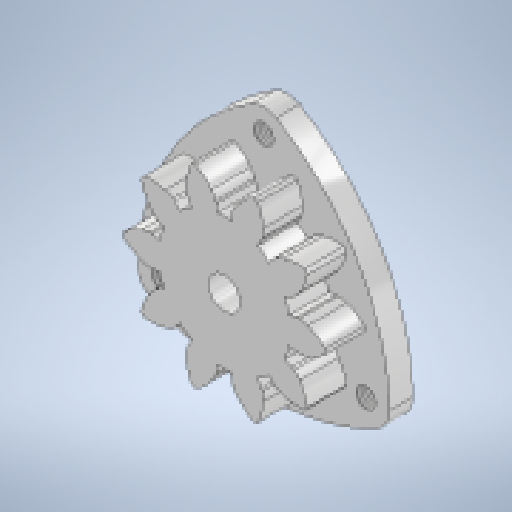
# Autodesk Inventor part: 多段ギアm2z10t8
Saved by Autodesk Inventor 2023 (Build 270158030, 158C)
## iProperties
Created: 2022-01-10
Part Number: 多段ギアm2z10t8
Material: アルミニウム 2014-T6
Document SubType Name: Modeling
Designer: acps
Density: 2.78927 g/cm^3
Appearance: サテン
Mass: 10.7159 g
Surface Area: 25.2572 cm^2
Volume: 3.84181 cm^3
Author: acps
Autodesk Inventor part; units mm, degrees
ref_plane "YZ Plane" through (0, 0, 0) normal (1, 0, 0) x (0, 1, 0)
ref_plane "XZ Plane" through (0, 0, 0) normal (0, 1, 0) x (-1, 0, 0)
ref_plane "XY Plane" through (0, 0, 0) normal (0, 0, 1) x (1, 0, 0)
sketch "Sketch1" plane through (0, 0, 0) normal (0, 0, 1) x (1, 0, 0)
  line L0 (0, -14) -> (0, 14)
  arc A0 (1.1104, 9.6344) -> (1.0261, 9.3407) centre (2.3502, 9.1195) ccw
  arc A1 (1.6598, 10.577) -> (1.1104, 9.6344) centre (4.6214, 8.2197) ccw
  arc A2 (3.6803, 12.3001) -> (1.6598, 10.577) centre (7.0807, 6.2665) ccw
  arc A3 (-4.7646, 8.4471) -> (-4.6602, 8.16) centre (-3.4589, 8.7593) ccw
  arc A4 (-4.8742, 9.5326) -> (-4.7646, 8.4471) centre (-1.0926, 9.3663) ccw
  arc A5 (-4.2524, 12.1142) -> (-4.8742, 9.5326) centre (2.0451, 9.2317) ccw
  arc A6 (-8.8197, 4.0333) -> (-8.5665, 3.8624) centre (-7.9469, 5.0533) ccw
  arc A7 (-9.5464, 4.847) -> (-8.8197, 4.0333) centre (-6.3893, 6.9353) ccw
  arc A8 (-10.5608, 7.3011) -> (-9.5464, 4.847) centre (-3.7717, 8.6706) ccw
  arc A9 (-9.506, -1.9211) -> (-9.2007, -1.9105) centre (-9.3994, -0.5829) ccw
  arc A10 (-10.5722, -1.6899) -> (-9.506, -1.9211) centre (-9.2455, 1.8552) ccw
  arc A11 (-12.8353, -0.3008) -> (-10.5722, -1.6899) centre (-8.1479, 4.7977) ccw
  arc A12 (-6.5613, -7.1417) -> (-6.3205, -6.9537) centre (-7.2617, -5.9964) ccw
  arc A13 (-7.5598, -7.5814) -> (-6.5613, -7.1417) centre (-8.5702, -3.9334) ccw
  arc A14 (-10.2072, -7.7878) -> (-7.5598, -7.5814) centre (-9.4118, -0.9078) ccw
  arc A15 (-1.1104, -9.6344) -> (-1.0261, -9.3407) centre (-2.3502, -9.1195) ccw
  arc A16 (-1.6598, -10.577) -> (-1.1104, -9.6344) centre (-4.6214, -8.2197) ccw
  arc A17 (-3.6803, -12.3001) -> (-1.6598, -10.577) centre (-7.0807, -6.2665) ccw
  arc A18 (4.7646, -8.4471) -> (4.6602, -8.16) centre (3.4589, -8.7593) ccw
  arc A19 (4.8742, -9.5326) -> (4.7646, -8.4471) centre (1.0926, -9.3663) ccw
  arc A20 (4.2524, -12.1142) -> (4.8742, -9.5326) centre (-2.0451, -9.2317) ccw
  arc A21 (8.8197, -4.0333) -> (8.5665, -3.8624) centre (7.9469, -5.0533) ccw
  arc A22 (9.5464, -4.847) -> (8.8197, -4.0333) centre (6.3893, -6.9353) ccw
  arc A23 (10.5608, -7.3011) -> (9.5464, -4.847) centre (3.7717, -8.6706) ccw
  arc A24 (9.506, 1.9211) -> (9.2007, 1.9105) centre (9.3994, 0.5829) ccw
  arc A25 (10.5722, 1.6899) -> (9.506, 1.9211) centre (9.2455, -1.8552) ccw
  arc A26 (12.8353, 0.3008) -> (10.5722, 1.6899) centre (8.1479, -4.7977) ccw
  arc A27 (6.5613, 7.1417) -> (6.3205, 6.9537) centre (7.2617, 5.9964) ccw
  arc A28 (7.5598, 7.5814) -> (6.5613, 7.1417) centre (8.5702, 3.9334) ccw
  arc A29 (10.2072, 7.7878) -> (7.5598, 7.5814) centre (9.4118, 0.9078) ccw
  arc A30 (-1.0261, 9.3407) -> (-1.1104, 9.6344) centre (-2.3502, 9.1195) ccw
  arc A31 (-1.1104, 9.6344) -> (-1.6598, 10.577) centre (-4.6214, 8.2197) ccw
  arc A32 (-1.6598, 10.577) -> (-3.6803, 12.3001) centre (-7.0807, 6.2665) ccw
  arc A33 (-6.3205, 6.9537) -> (-6.5613, 7.1417) centre (-7.2617, 5.9964) ccw
  arc A34 (-6.5613, 7.1417) -> (-7.5598, 7.5814) centre (-8.5702, 3.9334) ccw
  arc A35 (-7.5598, 7.5814) -> (-10.2072, 7.7878) centre (-9.4118, 0.9078) ccw
  arc A36 (-9.2007, 1.9105) -> (-9.506, 1.9211) centre (-9.3994, 0.5829) ccw
  arc A37 (-9.506, 1.9211) -> (-10.5722, 1.6899) centre (-9.2455, -1.8552) ccw
  arc A38 (-10.5722, 1.6899) -> (-12.8353, 0.3008) centre (-8.1479, -4.7977) ccw
  arc A39 (-8.5665, -3.8624) -> (-8.8197, -4.0333) centre (-7.9469, -5.0533) ccw
  arc A40 (-8.8197, -4.0333) -> (-9.5464, -4.847) centre (-6.3893, -6.9353) ccw
  arc A41 (-9.5464, -4.847) -> (-10.5608, -7.3011) centre (-3.7717, -8.6706) ccw
  arc A42 (-4.6602, -8.16) -> (-4.7646, -8.4471) centre (-3.4589, -8.7593) ccw
  arc A43 (-4.7646, -8.4471) -> (-4.8742, -9.5326) centre (-1.0926, -9.3663) ccw
  arc A44 (-4.8742, -9.5326) -> (-4.2524, -12.1142) centre (2.0451, -9.2317) ccw
  arc A45 (1.0261, -9.3407) -> (1.1104, -9.6344) centre (2.3502, -9.1195) ccw
  arc A46 (1.1104, -9.6344) -> (1.6598, -10.577) centre (4.6214, -8.2197) ccw
  arc A47 (1.6598, -10.577) -> (3.6803, -12.3001) centre (7.0807, -6.2665) ccw
  arc A48 (6.3205, -6.9537) -> (6.5613, -7.1417) centre (7.2617, -5.9964) ccw
  arc A49 (6.5613, -7.1417) -> (7.5598, -7.5814) centre (8.5702, -3.9334) ccw
  arc A50 (7.5598, -7.5814) -> (10.2072, -7.7878) centre (9.4118, -0.9078) ccw
  arc A51 (9.2007, -1.9105) -> (9.506, -1.9211) centre (9.3994, -0.5829) ccw
  arc A52 (9.506, -1.9211) -> (10.5722, -1.6899) centre (9.2455, 1.8552) ccw
  arc A53 (10.5722, -1.6899) -> (12.8353, -0.3008) centre (8.1479, 4.7977) ccw
  arc A54 (8.5665, 3.8624) -> (8.8197, 4.0333) centre (7.9469, 5.0533) ccw
  arc A55 (8.8197, 4.0333) -> (9.5464, 4.847) centre (6.3893, 6.9353) ccw
  arc A56 (9.5464, 4.847) -> (10.5608, 7.3011) centre (3.7717, 8.6706) ccw
  arc A57 (4.6602, 8.16) -> (4.7646, 8.4471) centre (3.4589, 8.7593) ccw
  arc A58 (4.7646, 8.4471) -> (4.8742, 9.5326) centre (1.0926, 9.3663) ccw
  arc A59 (4.8742, 9.5326) -> (4.2524, 12.1142) centre (-2.0451, 9.2317) ccw
  arc A60 (0.9173, 8.3498) -> (-0.9173, 8.3498) centre (0, 0) ccw
  arc A61 (-4.1658, 7.2943) -> (-5.65, 6.2159) centre (0, 0) ccw
  arc A62 (-7.6576, 3.4526) -> (-8.2246, 1.7078) centre (0, 0) ccw
  arc A63 (-8.2246, -1.7078) -> (-7.6576, -3.4526) centre (0, 0) ccw
  arc A64 (-5.65, -6.2159) -> (-4.1658, -7.2943) centre (0, 0) ccw
  arc A65 (-0.9173, -8.3498) -> (0.9173, -8.3498) centre (0, 0) ccw
  arc A66 (4.1658, -7.2943) -> (5.65, -6.2159) centre (0, 0) ccw
  arc A67 (7.6576, -3.4526) -> (8.2246, -1.7078) centre (0, 0) ccw
  arc A68 (8.2246, 1.7078) -> (7.6576, 3.4526) centre (0, 0) ccw
  arc A69 (5.65, 6.2159) -> (4.1658, 7.2943) centre (0, 0) ccw
  arc A70 (-3.6803, 12.3001) -> (-4.2524, 12.1142) centre (0, 0) ccw
  arc A71 (-10.2072, 7.7878) -> (-10.5608, 7.3011) centre (0, 0) ccw
  arc A72 (-12.8353, 0.3008) -> (-12.8353, -0.3008) centre (0, 0) ccw
  arc A73 (-10.5608, -7.3011) -> (-10.2072, -7.7878) centre (0, 0) ccw
  arc A74 (-4.2524, -12.1142) -> (-3.6803, -12.3001) centre (0, 0) ccw
  arc A75 (3.6803, -12.3001) -> (4.2524, -12.1142) centre (0, 0) ccw
  arc A76 (10.2072, -7.7878) -> (10.5608, -7.3011) centre (0, 0) ccw
  arc A77 (12.8353, -0.3008) -> (12.8353, 0.3008) centre (0, 0) ccw
  arc A78 (10.5608, 7.3011) -> (10.2072, 7.7878) centre (0, 0) ccw
  arc A79 (4.2524, 12.1142) -> (3.6803, 12.3001) centre (0, 0) ccw
  line L1 (0.9173, 8.3498) -> (1.0261, 9.3407)
  line L2 (-4.1658, 7.2943) -> (-4.6602, 8.16)
  line L3 (-7.6576, 3.4526) -> (-8.5665, 3.8624)
  line L4 (-8.2246, -1.7078) -> (-9.2007, -1.9105)
  line L5 (-5.65, -6.2159) -> (-6.3205, -6.9537)
  line L6 (-0.9173, -8.3498) -> (-1.0261, -9.3407)
  line L7 (4.1658, -7.2943) -> (4.6602, -8.16)
  line L8 (7.6576, -3.4526) -> (8.5665, -3.8624)
  line L9 (8.2246, 1.7078) -> (9.2007, 1.9105)
  line L10 (5.65, 6.2159) -> (6.3205, 6.9537)
  line L11 (-0.9173, 8.3498) -> (-1.0261, 9.3407)
  line L12 (-5.65, 6.2159) -> (-6.3205, 6.9537)
  line L13 (-8.2246, 1.7078) -> (-9.2007, 1.9105)
  line L14 (-7.6576, -3.4526) -> (-8.5665, -3.8624)
  line L15 (-4.1658, -7.2943) -> (-4.6602, -8.16)
  line L16 (0.9173, -8.3498) -> (1.0261, -9.3407)
  line L17 (5.65, -6.2159) -> (6.3205, -6.9537)
  line L18 (8.2246, -1.7078) -> (9.2007, -1.9105)
  line L19 (7.6576, 3.4526) -> (8.5665, 3.8624)
  line L20 (4.1658, 7.2943) -> (4.6602, 8.16)
  line L21 (-14.8388, 0) -> (14.8388, 0)
  line L22 (0, -14.8388) -> (0, 14.8388)
  circle A80 centre (0, 0) radius 2
  dimension "d32" = 4
  constraints: 160 point on circle, 81 centre point, 46 end point, 1 coincident
  measures "d32" diameter of A80
extrude "Extrusion1" add sketch "Sketch1" along normal blind 5 contours A65 L6 A15 A16 A17 A74 A44 A43 A42 L15 A64 L5 A12 A13 A14 A73 A41 A40 A39 L14 A63 L4 A9 A10 A11 A72 L21 A80 L0 | L0 A80 L21 A77 A53 A52 A51 L18 A67 L8 A21 A22 A23 A76 A50 A49 A48 L17 A66 L7 A18 A19 A20 A75 A47 A46 A45 L16 A65 | L21 A72 A38 A37 A36 L13 A62 L3 A6 A7 A8 A71 A35 A34 A33 L12 A61 L2 A3 A4 A5 A70 A32 A31 A30 L11 A60 L0 A80 | A80 L0 A60 L1 A0 A1 A2 A79 A59 A58 A57 L20 A69 L10 A27 A28 A29 A78 A56 A55 A54 L19 A68 L9 A24 A25 A26 A77 L21
sketch "Sketch3" plane through (0, 0, 0) normal (0, 0, -1) x (-1, 0, 0)
  circle A0 centre (-12.9904, -7.5) radius 1.25
  circle A1 centre (12.9904, -7.5) radius 1.25
  circle A2 centre (0, 15) radius 1.25
  circle A3 centre (0, 0) radius 20.05 construction
  circle A4 centre (0, 0) radius 18.25 construction
  circle A5 centre (-12.9904, -7.5) radius 3.25 construction
  circle A6 centre (-12.9904, -7.5) radius 3
  circle A7 centre (12.9904, -7.5) radius 3
  circle A8 centre (0, 15) radius 3
  arc A9 (-1.5559, 17.565) -> (-15.9897, -7.435) centre (14.0033, -8.0848) ccw
  arc A10 (-14.4338, -10.13) -> (14.4338, -10.13) centre (0, 16.1696) ccw
  arc A11 (15.9897, -7.435) -> (1.5559, 17.565) centre (-14.0033, -8.0848) ccw
  circle A12 centre (0, 0) radius 2
  point P0 (15.9897, -7.435)
  point P1 (1.5559, 17.565)
  point P2 (-14.4338, -10.13)
  point P3 (14.4338, -10.13)
  dimension "d14" = 6
  dimension "d18" = 6
  dimension "d3" = 2.5
  dimension "d6" = 360
  dimension "d9" = 40.1
  dimension "d10" = 36.5
  dimension "d11" = 6.5
  dimension "d17" = 6
  dimension "d19" = 30
  dimension "d22" = 360
  dimension "d33" = 4
  constraints: 11 centre point, 7 coincident, 6 point on circle, 1 horizontal alignment, 1 tangent, 28 other
  measures "d3" diameter of A0
  measures "d9" diameter of A3
  measures "d10" diameter of A4
  measures "d11" diameter of A5
  measures "d17" diameter of A7
  measures "d19" radius of A9
  measures "d33" diameter of A12
extrude "Extrusion2" add sketch "Sketch3" along normal blind 3
thread "Thread1" size "M3x0.5" class "6H" standard "ANSI Metric M Profile" full length
thread "Thread2" size "M3x0.5" class "6H" standard "ANSI Metric M Profile" full length
thread "Thread3" size "M3x0.5" class "6H" standard "ANSI Metric M Profile" full length
body "Solid1"
